z_guide_holder_right (Autodesk Fusion 360 design; units mm, degrees)
Autodesk Fusion 360 part; units mm, degrees
note: some values were not read from the file. Set by a fixed rule: which sketch regions a step uses.
sketch "Sketch1" plane through (0, 0, 0) normal (0, 0, 1) x (1, 0, 0)
  circle A0 centre (0, 0) radius 5
  circle A1 centre (-17, 0) radius 4
  line L0 (-27, 29.15) -> (-27, -10)
  line L1 (-27, -10) -> (10, -10)
  line L2 (10, -10) -> (10, 29.15)
  line L3 (10, 29.15) -> (50, 29.15)
  line L4 (50, 29.15) -> (50, 59.15)
  line L5 (50, 59.15) -> (-5, 59.15)
  line L6 (-5, 59.15) -> (-27, 29.15)
  circle A2 centre (14.15, 44.15) radius 4.25
  circle A3 centre (40, 44.15) radius 2.6
  dimension "d3" = 10
  dimension "d4" = 8
  dimension "d5" = 17
  dimension "d6" = 10
  dimension "d7" = 10
  dimension "d8" = 10
  dimension "d9" = 30
  dimension "d10" = 29.15
  dimension "d11" = 15
  dimension "d12" = 40
  dimension "d15" = 8.5
  dimension "d16" = 15
  dimension "d17" = 4.15
  dimension "d18" = 10
  dimension "d30" = 5.2
  constraint coincident A0.centre origin
  constraint horizontal A0.centre A1.centre
  constraint vertical L0
  constraint perpendicular L0 L1
  constraint perpendicular L1 L2
  constraint perpendicular L2 L3
  constraint perpendicular L3 L4
  constraint perpendicular L4 L5
  constraint horizontal L0.start L2.end
  constraint horizontal A2.centre A3.centre
  measures "d3" diameter of A0
  measures "d4" diameter of A1
  measures "d5" distance of A0.centre A1.centre
  measures "d6" distance of A1.centre L1
  measures "d7" distance of A1.centre L0
  measures "d8" distance of A0.centre L2
  measures "d9" distance of L3 L5
  measures "d10" distance of A0.centre L3
  measures "d11" horizontal distance of L2.end L5.end
  measures "d12" distance of L2.end L3.end
  measures "d15" diameter of A2
  measures "d16" distance of L3 A2.centre
  measures "d17" distance of L2 A2.centre
  measures "d18" distance of L4 A3.centre
  measures "d30" diameter of A3
extrude "Extrude1" add sketch "Sketch1" along normal blind 6 makes body 1
sketch "Sketch2" plane through (0, 0, 0) normal (0, 0, -1) x (1, 0, 0)
  circle A0 centre (-17, 0) radius 4
  circle A1 centre (14.15, -44.15) radius 4.25
  circle A2 centre (0, 0) radius 5
  circle A3 centre (40, -44.15) radius 2.6
  line L0 (-27, -29.15) -> (-5, -59.15)
  line L1 (-5, -59.15) -> (50, -59.15)
  line L2 (50, -59.15) -> (50, -29.15)
  line L3 (50, -29.15) -> (10, -29.15)
  line L4 (10, -29.15) -> (10, 10)
  line L5 (10, 10) -> (-27, 10)
  line L6 (-27, 10) -> (-27, -29.15)
  line L7 (10, -29.15) -> (-27, -29.15)
  line L8 (-27, -26.15) -> (10, -26.15)
  line L9 (-0.85, -29.15) -> (-0.85, -59.15)
  line L10 (-3.85, -60.7182) -> (-3.85, -29.15)
  dimension "d19" = 3
  dimension "d20" = 0.85
  dimension "d21" = 3
  constraint coincident L3.end L4.start
  constraint coincident L0.start L6.end
  constraint coincident L6 L8.start
  constraint coincident L4 L8.end
  constraint perpendicular L4 L8
  constraint coincident L7 L9.start
  constraint coincident L1 L9.end
  constraint perpendicular L1 L9
  constraint coincident L0 L10.start
  constraint coincident L7 L10.end
  constraint perpendicular L7 L10
  measures "d19" distance of L7 L8
  measures "d20" distance of A2.centre L9
  measures "d21" distance of L9 L10
extrude "Extrude2" add sketch "Sketch2" along normal blind 2 contours L0 L1 L7 L10 | L4 L6 L7 L8 | L1 L7 L9 L10 bodies 1
fillet "Fillet1" radius 10 1 edges at (10, 29.15, 3) on bodies 1
fillet "Fillet2" radius 3 6 edges at (50, 29.15, 3) (50, 59.15, 3) (10, -10, 3) (-27, -10, 3) (-27, 29.15, 2) (-5, 59.15, 2) on bodies 1
mirror "Mirror1" about plane through (50, 29.15, 0) normal (1, 0, 0) of bodies 1 makes body 2
hidden bodies 1
equation "d16 = d9 / 2"
equation "d21 = d19"
